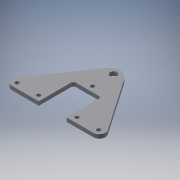
# Autodesk Inventor part: Corpo_Suporte_4_Cabos_Modelo3
Saved by Autodesk Inventor 2018 (Build 220112000, 112)
## iProperties
Created: 2021-08-02
Part Number: Corpo_Suporte_4_Cabos_Modelo3
Material: Generic
Document SubType Name: Modeling
Designer: L08619
Density: 1 g/cm^3
Appearance: Default
Author: L08619
Autodesk Inventor part; units mm, degrees
ref_plane "YZ Plane" through (0, 0, 0) normal (1, 0, 0) x (0, 1, 0)
ref_plane "XZ Plane" through (0, 0, 0) normal (0, 1, 0) x (-1, 0, 0)
ref_plane "XY Plane" through (0, 0, 0) normal (0, 0, 1) x (1, 0, 0)
sketch "Sketch1" plane through (0, 0, 0) normal (0, 0, 1) x (1, 0, 0)
  circle A0 centre (0, 0) radius 20
  circle A1 centre (0, -120) radius 11
  circle A2 centre (-235, -320) radius 11
  circle A3 centre (235, -320) radius 11
  arc A4 (233.6625, -350) -> (260.9808, -293.1206) centre (233.6625, -315) ccw
  line L0 (260.9808, -293.1206) -> (60, 0)
  line L1 (0, 0) -> (0, -429.6945)
  arc A5 (-260.9808, -293.1206) -> (-233.6625, -350) centre (-233.6625, -315) ccw
  line L2 (-260.9808, -293.1206) -> (-60, 0)
  spline S0 degree 2 poles (-60, 0) (0.0011, 80.0234) (60, 0) knots 0 0 0 1 1 1
  line L3 (0, -150) -> (70, -150)
  line L4 (-80, -240) -> (-80, -160)
  line L5 (-70, -150) -> (0, -150)
  line L6 (-80, -160) -> (-70, -150)
  line L7 (80, -160) -> (70, -150)
  line L8 (-80, -160) -> (-80, -350)
  line L9 (80, -160) -> (80, -350)
  line L10 (-233.6625, -350) -> (-80, -350)
  line L11 (80, -350) -> (233.6625, -350)
  circle A6 centre (-110, -320) radius 11
  circle A7 centre (110, -320) radius 11
  point P0 (0.0008, 40.0117)
  point P1 (80, -150)
  point P2 (60, -250)
  point P3 (-80, -150)
  dimension "d0" = 40
  dimension "d1" = 22
  dimension "d3" = 22
  dimension "d4" = 22
  dimension "d5" = 120
  dimension "d9" = 35
  dimension "d14" = 60
  dimension "d15" = 60
  dimension "d16" = 80
  dimension "d19" = 10
  dimension "d20" = 10
  dimension "d21" = 10
  dimension "d22" = 10
  dimension "d27" = 30
  dimension "d30" = 22
  dimension "d31" = 22
  dimension "d32" = 30
  dimension "d33" = 30
  dimension "d36" = 160
  constraints: 24 end point, 8 centre point, 6 point on line, 4 point on circle, 3 horizontal, 3 symmetric about line, 2 tangent, 1 coincident, 1 perpendicular, 1 vertical, 6 other
  measures "d0" diameter of A0
  measures "d1" diameter of A1
  measures "d3" diameter of A2
  measures "d4" diameter of A3
  measures "d5" distance of A1.centre point (0, 0)
  measures "d9" radius of A4
  measures "d14" distance of L2.end L1.start
  measures "d15" distance of L0.end point (0, 0)
  measures "d16" distance of L3.start point (80, -150)
  measures "d19" distance of L4.end point (-80, -150)
  measures "d20" distance of L5.start point (-80, -150)
  measures "d21" distance of L7.start point (80, -150)
  measures "d22" distance of L3.end point (80, -150)
  measures "d27" distance from line of L5 A1.centre
  measures "d30" diameter of A6
  measures "d31" diameter of A7
  measures "d32" distance from line of L8 A6.centre
  measures "d33" distance from line of L9 A7.centre
  measures "d36" distance between parallel lines of L8 L9
extrude "Extrusion2" add sketch "Sketch1" along normal mid plane 22.22
equation "\"d20\" = d19"
equation "\"d21\" = d19"
equation "\"d22\" = d21"
body "Solid2"
